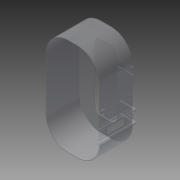
# Autodesk Inventor part: coil_former_mold_new
Saved by Autodesk Inventor 2014 SP1 (Build 180222100, 222)
## iProperties
Created: 2016-09-07
Part Number: coil_former_mold_new
Material: Polycarbonate, Clear
Document SubType Name: Modeling
Designer: tguillod
Density: 1.2 g/cm^3
Appearance: Polycarbonate - Clear
Author: tguillod
Autodesk Inventor part; units mm, degrees
ref_plane "YZ Plane" through (0, 0, 0) normal (1, 0, 0) x (0, 1, 0)
ref_plane "XZ Plane" through (0, 0, 0) normal (0, 1, 0) x (-1, 0, 0)
ref_plane "XY Plane" through (0, 0, 0) normal (0, 0, 1) x (1, 0, 0)
sketch "Sketch1" plane through (0, 0, 0) normal (0, 0, 1) x (1, 0, 0)
  line L0 (0, 0) -> (1, 0)
  line L1 (1, 0) -> (1, 57.5)
  line L2 (1, 57.5) -> (0, 57.5)
  line L3 (0, 57.5) -> (0, 0)
  line L4 (1, 57.5) -> (-26, 57.5)
  line L5 (-26, 57.5) -> (-26, 58.5)
  line L6 (-26, 58.5) -> (1, 58.5)
  line L7 (1, 58.5) -> (1, 57.5)
  dimension "d90" = 10
  dimension "d1" = 1
  dimension "d7" = 1
  dimension "d8" = 27
  dimension "d9" = 58.5
  constraints: 16 end point, 4 parallel, 2 horizontal, 2 perpendicular
  measures "d1" distance of L0.start L0.end
  measures "d7" distance of L6.end L1.end
  measures "d8" distance of L5.end L6.end
  measures "d9" distance from line of L0.end L6
sketch "Sketch2" plane through (0, 0, 0) normal (0, 1, 0) x (-1, 0, 0)
  line L0 (0, 0) -> (0, 46.75)
  line L1 (37, 83.75) -> (45.5, 83.75)
  arc A0 (37, 83.75) -> (0, 46.75) centre (37, 46.75) ccw
  point P0 (0, 83.75)
  dimension "d3" = 83.75
  dimension "d4" = 45.5
  dimension "d5" = 37
  constraints: 4 end point, 2 point on circle, 2 point on line, 2 tangent, 1 centre point, 1 perpendicular, 1 vertical
  measures "d3" distance of L0.start point (0, 83.75)
  measures "d4" distance of point (0, 83.75) L1.end
  measures "d5" radius of A0
sweep "Sweep1" add profiles "Sketch1" path "Sketch2" path curves L0 A0 L1
mirror "Mirror1" about plane through (0.5, 28.75, 0) normal (0, 0, -1)
mirror "Mirror2" about plane through (-45.5, 28.75, -84.25) normal (-1, 0, 0)
sketch "Sketch3" plane through (-26, 58.5, 0) normal (0, 1, 0) x (1, 0, 0)
  line L0 (27, 0) -> (0, 0) projected
  line L1 (0, 0) -> (0, -46.75) projected
  line L2 (0, -40) -> (10, -40)
  line L3 (10, -40) -> (10, -30)
  line L4 (10, -30) -> (0, -30)
  line L5 (0, -30) -> (0, -40)
  point P0 (26, 0)
  dimension "d10" = 30
  dimension "d11" = 10
  dimension "d12" = 10
  constraints: 8 end point, 2 parallel, 1 collinear, 1 horizontal, 1 perpendicular
  measures "d10" distance between parallel lines of L0 L4
  measures "d11" distance of L2.end L3.end
  measures "d12" distance of L2.start L2.end
extrude "Extrusion1" cut sketch "Sketch3" against normal blind 10
sketch "Sketch4" plane through (1, 58.5, 46.75) normal (0, 1, 0) x (1, 0, 0)
  line L0 (0, 93.5) -> (0, 0) projected
  line L1 (-7, 80.25) -> (-2, 80.25)
  line L2 (-2, 80.25) -> (-2, 76.25)
  line L3 (-2, 76.25) -> (-7, 76.25)
  line L4 (-7, 76.25) -> (-7, 80.25)
  point P0 (-1, 46.75)
  dimension "d16" = 5
  dimension "d17" = 4
  dimension "d18" = 2
  dimension "d19" = 29.5
  constraints: 8 end point, 2 parallel, 1 horizontal, 1 perpendicular
  measures "d16" distance of L1.start L1.end
  measures "d17" distance of L1.end L2.end
  measures "d18" distance between parallel lines of L0 L2
  measures "d19" distance from line of point (-1, 46.75) L3
extrude "Extrusion2" cut sketch "Sketch4" against normal blind 10
fillet "Fillet1" radius 3 2 edges at (-16, 58, 40) (-16, 58, 30)
sketch "Sketch7" plane through (1, 58.5, 46.75) normal (0, 1, 0) x (1, 0, 0)
  line L0 (-7, 80.25) -> (-2, 80.25) projected
  line L1 (-2, 76.25) -> (-7, 76.25) projected
  line L2 (-27, 93.5) -> (-27, 16.75) projected
  line L3 (0, 93.5) -> (0, 0) projected
  line L4 (-24, 88.25) -> (0, 88.25)
  line L5 (0, 88.25) -> (0, 87.25)
  line L6 (0, 87.25) -> (-24, 87.25)
  line L7 (-24, 87.25) -> (-24, 88.25)
  line L8 (0, 68.25) -> (-24, 68.25)
  line L9 (-24, 68.25) -> (-24, 69.25)
  line L10 (-24, 69.25) -> (0, 69.25)
  line L11 (0, 69.25) -> (0, 68.25)
  point P0 (-1, 46.75)
  dimension "d38" = 1
  dimension "d39" = 1
  dimension "d40" = 7
  dimension "d41" = 7
  dimension "d42" = 3
  constraints: 16 end point, 4 parallel, 2 horizontal, 2 perpendicular, 2 point on line, 1 collinear
  measures "d38" distance of L6.end L4.start
  measures "d39" distance of L8.end L9.end
  measures "d40" distance between parallel lines of L1 L10
  measures "d41" distance between parallel lines of L6 L0
  measures "d42" distance between parallel lines of L2 L7
extrude "Extrusion5" add sketch "Sketch7" along normal blind 3
sketch "Sketch8" plane through (1, 58.5, -41.5) normal (0, 0, -1) x (-1, 0, 0)
  line L0 (24, 0) -> (24, 3) projected
  line L1 (0, 3) -> (24, 3)
  line L2 (24, 3) -> (24, 2)
  line L3 (24, 2) -> (0, 2)
  line L4 (0, 2) -> (0, 3)
  point P0 (1, -58.5)
  dimension "d45" = 1
  constraints: 8 end point, 2 parallel, 1 horizontal, 1 perpendicular, 1 point on line
  measures "d45" distance of L1.end L2.end
extrude "Extrusion6" add sketch "Sketch8" along normal blind 1
sketch "Sketch9" plane through (-23, 58.5, -21.5) normal (0, 0, 1) x (1, 0, 0)
  line L0 (24, 0) -> (24, 3) projected
  line L1 (0, 3) -> (24, 3)
  line L2 (24, 3) -> (24, 2)
  line L3 (24, 2) -> (0, 2)
  line L4 (0, 2) -> (0, 3)
  point P0 (23, -58.5)
  dimension "d48" = 1
  constraints: 8 end point, 2 parallel, 1 horizontal, 1 perpendicular, 1 point on line
  measures "d48" distance of L1.end L2.end
extrude "Extrusion7" add sketch "Sketch9" along normal blind 1
sketch "Sketch10" plane through (1, 0, 46.75) normal (1, 0, 0) x (0, 0, -1)
  line L0 (68.25, 58.5) -> (68.25, 60.5) projected
  line L1 (93.5, 0) -> (0, 0) projected
  line L2 (69.25, 61.5) -> (68.25, 61.5)
  line L3 (68.25, 61.5) -> (68.25, -4)
  line L4 (68.25, -4) -> (69.25, -4)
  line L5 (69.25, -4) -> (69.25, 61.5)
  line L6 (87.25, 61.5) -> (88.25, 61.5)
  line L7 (88.25, 61.5) -> (88.25, -4)
  line L8 (88.25, -4) -> (87.25, -4)
  line L9 (87.25, -4) -> (87.25, 61.5)
  point P0 (88.25, 60.5)
  point P1 (46.75, 0)
  dimension "d51" = 4
  constraints: 16 end point, 4 parallel, 2 collinear, 2 horizontal, 2 perpendicular, 2 point on line
  measures "d51" distance between parallel lines of L1 L4
extrude "Extrusion8" add sketch "Sketch10" along normal blind 3
sketch "Sketch12" plane through (-23, 58.5, -21.5) normal (0, 0, 1) x (1, 0, 0)
  line L0 (24, -58.5) -> (24, -62.5) projected
  line L1 (24, -62.5) -> (27, -62.5) projected
  line L2 (27, 3) -> (27, -62.5) projected
  line L3 (24, 3) -> (27, 3) projected
  line L4 (24, 2) -> (24, 3) projected
  line L5 (24, -62.5) -> (24, -61.5)
  line L6 (26, -61.5) -> (26, 2)
  line L7 (26, 2) -> (24, 2)
  line L8 (24, 3) -> (27, 3)
  line L9 (27, -62.5) -> (27, 3)
  line L10 (27, -62.5) -> (24, -62.5)
  line L11 (24, -61.5) -> (26, -61.5)
  point P0 (23, -58.5)
  dimension "d56" = 1
  dimension "d57" = 1
  constraints: 14 end point, 3 collinear, 2 parallel, 1 perpendicular, 1 point on line
  measures "d56" distance between parallel lines of L9 L6
  measures "d57" distance between parallel lines of L1 L11
extrude "Extrusion9" add sketch "Sketch12" along normal blind 1
sketch "Sketch13" plane through (1, 58.5, -41.5) normal (0, 0, -1) x (-1, 0, 0)
  line L0 (24, 2) -> (0, 2) projected
  line L1 (0, 3) -> (0, 2) projected
  line L2 (0, 3) -> (-3, 3) projected
  line L3 (-3, -62.5) -> (-3, 3) projected
  line L4 (0, -62.5) -> (-3, -62.5) projected
  line L5 (0, -62.5) -> (0, -58.5) projected
  line L6 (24, 0) -> (0, 0) projected
  line L7 (0, 2) -> (0, 3)
  line L8 (-3, 3) -> (0, 3)
  line L9 (-3, 3) -> (-3, -62.5)
  line L10 (-3, -62.5) -> (0, -62.5)
  line L11 (0, -62.5) -> (0, -61.5)
  line L12 (-2, -61.5) -> (0, -61.5)
  line L13 (-2, -61.5) -> (-2, 2)
  line L14 (-2, 2) -> (0, 2)
  point P0 (1, -58.5)
  dimension "d60" = 1
  dimension "d61" = 1
  constraints: 16 end point, 4 perpendicular, 3 collinear, 1 point on line
  measures "d60" distance between parallel lines of L10 L12
  measures "d61" distance between parallel lines of L3 L13
extrude "Extrusion10" add sketch "Sketch13" along normal blind 1
sketch "Sketch16" plane through (1, 58.5, -22.5) normal (1, 0, 0) x (0, 0, -1)
  line L0 (0, 0) -> (0, -58.5) projected
  line L1 (18, -58.5) -> (0, -58.5) projected
  line L2 (18, -58.5) -> (18, 0) projected
  line L3 (18, 0) -> (0, 0) projected
  line L4 (3, 0) -> (4, 0)
  line L5 (4, 0) -> (4, -12)
  line L6 (4, -12) -> (3, -12)
  line L7 (3, -12) -> (3, 0)
  line L8 (15, 0) -> (14, 0)
  line L9 (14, 0) -> (14, -12)
  line L10 (14, -12) -> (15, -12)
  line L11 (15, -12) -> (15, 0)
  line L12 (3, -58.5) -> (4, -58.5)
  line L13 (4, -58.5) -> (4, -47.5)
  line L14 (4, -47.5) -> (3, -47.5)
  line L15 (3, -47.5) -> (3, -58.5)
  line L16 (15, -58.5) -> (14, -58.5)
  line L17 (14, -58.5) -> (14, -47.5)
  line L18 (14, -47.5) -> (15, -47.5)
  line L19 (15, -47.5) -> (15, -58.5)
  line L20 (3, -12) -> (15, -12)
  line L21 (15, -12) -> (15, -13)
  line L22 (15, -13) -> (3, -13)
  line L23 (3, -13) -> (3, -12)
  line L24 (3, -47.5) -> (15, -47.5)
  line L25 (15, -47.5) -> (15, -46.5)
  line L26 (15, -46.5) -> (3, -46.5)
  line L27 (3, -46.5) -> (3, -47.5)
  point P0 (-22.5, -58.5)
  dimension "d77" = 1
  dimension "d78" = 1
  dimension "d79" = 12
  dimension "d80" = 11
  dimension "d81" = 1
  dimension "d82" = 1
  dimension "d83" = 1
  dimension "d84" = 1
  dimension "d85" = 3
  dimension "d86" = 3
  dimension "d87" = 10
  dimension "d88" = 3
  dimension "d89" = 3
  dimension "d90" = 10
  constraints: 48 end point, 12 parallel, 6 horizontal, 6 perpendicular, 4 collinear, 4 point on line
  measures "d77" distance of L5.end L6.end
  measures "d78" distance of L9.end L10.end
  measures "d79" distance of L10.end L8.start
  measures "d80" distance of L18.end L16.start
  measures "d81" distance of L17.end L18.end
  measures "d82" distance of L13.end L14.end
  measures "d83" distance of L26.end L14.end
  measures "d84" distance of L22.end L6.end
  measures "d85" distance between parallel lines of L0 L7
  measures "d86" distance between parallel lines of L11 L2
  measures "d87" distance between parallel lines of L9 L5
  measures "d88" distance between parallel lines of L0 L15
  measures "d89" distance between parallel lines of L19 L2
  measures "d90" distance between parallel lines of L17 L13
extrude "Extrusion13" add sketch "Sketch16" along normal blind 1 contours L3 L5 L6 L7 | L15 L14 L13 L1 | L6 L20 L10 L21 L22 L23 | L27 L26 L25 L18 L24 L14 | L3 L11 L10 L9 | L17 L18 L19 L1
sketch "Sketch17" plane through (-54, 0, -84.75) normal (0, -1, 0) x (1, 0, 0)
  line L0 (56, 59.25) -> (55, 59.25)
  line L1 (55, 59.25) -> (55, 58.25)
  line L2 (55, 58.25) -> (56, 58.25)
  line L3 (56, 58.25) -> (56, 59.25)
  line L4 (56, 48.25) -> (55, 48.25)
  line L5 (55, 48.25) -> (55, 47.25)
  line L6 (55, 47.25) -> (56, 47.25)
  line L7 (56, 47.25) -> (56, 48.25)
  point P0 (54, 84.75)
  constraints: 16 end point, 4 parallel, 2 horizontal, 2 perpendicular
extrude "Extrusion14" add sketch "Sketch17" along normal blind 1
sketch "Sketch18" plane through (-54, 58.5, -84.75) normal (0, 1, 0) x (1, 0, 0)
  line L0 (55, -63.25) -> (55, -131.5) projected
  line L1 (28, -114.75) -> (55, -114.75)
  line L2 (55, -114.75) -> (55, -113.75)
  line L3 (55, -113.75) -> (28, -113.75)
  line L4 (28, -113.75) -> (28, -114.75)
  line L5 (28, -124.75) -> (55, -124.75)
  line L6 (55, -124.75) -> (55, -125.75)
  line L7 (55, -125.75) -> (28, -125.75)
  line L8 (28, -125.75) -> (28, -124.75)
  point P0 (54, -84.75)
  dimension "d95" = 1
  dimension "d96" = 1
  constraints: 16 end point, 4 parallel, 2 horizontal, 2 perpendicular, 2 point on line
  measures "d95" distance of L1.end L2.end
  measures "d96" distance between parallel lines of L5 L7
extrude "Extrusion15" add sketch "Sketch18" along normal blind 1
sketch "Sketch20" plane through (1, 0, 46.75) normal (1, 0, 0) x (0, 0, -1)
  line L0 (68.25, 58.5) -> (17.75, 58.5) projected
  line L1 (0, 0) -> (0, 58.5) projected
  line L2 (68.25, 0) -> (0, 0) projected
  line L3 (42.75, 55.5) -> (50.75, 55.5)
  line L4 (50.75, 55.5) -> (50.75, 48.5)
  line L5 (50.75, 48.5) -> (42.75, 48.5)
  line L6 (42.75, 48.5) -> (42.75, 55.5)
  line L7 (42.75, 9) -> (50.75, 9)
  line L8 (50.75, 9) -> (50.75, 2)
  line L9 (50.75, 2) -> (42.75, 2)
  line L10 (42.75, 2) -> (42.75, 9)
  line L11 (43.75, 54.5) -> (49.75, 54.5)
  line L12 (49.75, 54.5) -> (49.75, 49.5)
  line L13 (49.75, 49.5) -> (43.75, 49.5)
  line L14 (43.75, 49.5) -> (43.75, 54.5)
  line L15 (43.75, 8) -> (49.75, 8)
  line L16 (49.75, 8) -> (49.75, 3)
  line L17 (49.75, 3) -> (43.75, 3)
  line L18 (43.75, 3) -> (43.75, 8)
  point P0 (46.75, 0)
  dimension "d112" = 8
  dimension "d113" = 7
  dimension "d114" = 7
  dimension "d116" = 2
  dimension "d117" = 3
  dimension "d118" = 42.75
  dimension "d119" = 1
  dimension "d120" = 1
  dimension "d121" = 1
  dimension "d122" = 1
  dimension "d123" = 1
  dimension "d124" = 1
  dimension "d125" = 1
  dimension "d126" = 1
  constraints: 32 end point, 8 parallel, 4 horizontal, 4 perpendicular, 2 collinear
  measures "d112" distance of L3.start L3.end
  measures "d113" distance of L3.end L4.end
  measures "d114" distance of L7.end L8.end
  measures "d116" distance between parallel lines of L2 L9
  measures "d117" distance between parallel lines of L0 L3
  measures "d118" distance between parallel lines of L1 L6
  measures "d119" distance between parallel lines of L3 L11
  measures "d120" distance between parallel lines of L6 L14
  measures "d121" distance between parallel lines of L5 L13
  measures "d122" distance between parallel lines of L4 L12
  measures "d123" distance between parallel lines of L7 L15
  measures "d124" distance between parallel lines of L8 L16
  measures "d125" distance between parallel lines of L17 L9
  measures "d126" distance between parallel lines of L10 L18
extrude "Extrusion17" add sketch "Sketch20" along normal blind 1
fillet "Fillet7" radius 1 14 edges at (-45.5, 58.5, -84.75) (-80.8701, 58.5, -73.6201) (-92, 58.5, 0) (-80.8701, 58.5, 73.6201) (-45.5, 58.5, 84.75) (-10.1299, 58.5, 73.6201) (1, 58.5, 43.875) (1, 58.5, -44.125) (-10.1299, 58.5, -73.6201) (1, 58.5, 35) (1, 58.5, 3.75) (1, 58.5, -24) (1, 58.5, -31.5) (1, 58.5, -39)
fillet "Fillet8" radius 1 4 edges at (3, 60.5, -42) (3, -3, -42) (3, 60.5, -21) (3, -3, -21)
sketch "Sketch23" plane through (1, 0, 46.75) normal (-1, 0, 0) x (0, 0, 1)
  line L0 (-88.25, 0) -> (-87.25, 0) projected
  line L1 (-88.25, -3) -> (-88.25, 0) projected
  line L2 (-88.25, -3) -> (-89.25, -3) projected
  line L3 (-89.25, -4) -> (-89.25, -3) projected
  line L4 (-87.25, -4) -> (-89.25, -4) projected
  line L5 (-87.25, 0) -> (-87.25, -4) projected
  line L6 (-69.25, 0) -> (-68.25, 0) projected
  line L7 (-69.25, -4) -> (-69.25, 0) projected
  line L8 (-69.25, -4) -> (-67.25, -4) projected
  line L9 (-67.25, -3) -> (-67.25, -4) projected
  line L10 (-68.25, -3) -> (-67.25, -3) projected
  line L11 (-68.25, 0) -> (-68.25, -3) projected
  line L12 (-89.25, -3) -> (-87.25, -3)
  line L13 (-87.25, -3) -> (-87.25, -4)
  line L14 (-87.25, -4) -> (-89.25, -4)
  line L15 (-89.25, -4) -> (-89.25, -3)
  line L16 (-87.25, -3) -> (-88.25, -3)
  line L17 (-88.25, -3) -> (-88.25, 0)
  line L18 (-88.25, 0) -> (-87.25, 0)
  line L19 (-87.25, 0) -> (-87.25, -3)
  line L20 (-88.25, 0) -> (-89.25, 0)
  line L21 (-89.25, 0) -> (-89.25, -1)
  line L22 (-89.25, -1) -> (-88.25, -1)
  line L23 (-88.25, -1) -> (-88.25, 0)
  line L24 (-67.25, -3) -> (-69.25, -3)
  line L25 (-69.25, -3) -> (-69.25, -4)
  line L26 (-69.25, -4) -> (-67.25, -4)
  line L27 (-67.25, -4) -> (-67.25, -3)
  line L28 (-68.25, -3) -> (-69.25, -3)
  line L29 (-69.25, -3) -> (-69.25, 0)
  line L30 (-69.25, 0) -> (-68.25, 0)
  line L31 (-68.25, 0) -> (-68.25, -3)
  line L32 (-68.25, 0) -> (-67.25, 0)
  line L33 (-67.25, 0) -> (-67.25, -1)
  line L34 (-67.25, -1) -> (-68.25, -1)
  line L35 (-68.25, -1) -> (-68.25, 0)
  point P0 (-46.75, 0)
  constraints: 48 end point, 12 parallel, 6 horizontal, 6 perpendicular, 4 collinear
extrude "Extrusion19" add sketch "Sketch23" along normal blind 2
fillet "Fillet10" radius 1 2 edges at (1, -1, -42) (1, -1, -21)
fillet "Fillet11" radius 1 20 edges at (-0.5, -1, -41.5) (1, 28.75, -41.5) (0.7071, 58.2071, -41.5) (-11.5, 58.5, -41.5) (0.7071, -0.7071, -41.5) (2.7071, -2.7071, -41.5) (3, 28.75, -41.5) (2.7071, 60.2071, -41.5) (-10.5, 60.5, -41.5) (0.5, -3, -41.5) (2.7071, -2.7071, -21.5) (3, 28.75, -21.5) (2.7071, 60.2071, -21.5) (-10.5, 60.5, -21.5) (0.5, -3, -21.5) (1, 28.75, -21.5) (0.7071, 58.2071, -21.5) (-11.5, 58.5, -21.5) (-0.5, -1, -21.5) (0.7071, -0.7071, -21.5)
sketch "Sketch24" plane through (0, 0, -42.5) normal (0, 0, -1) x (-1, 0, 0)
  line L0 (23, 60.5) -> (23, 61.5) projected
  line L1 (23, 61.5) -> (-4, 61.5) projected
  line L2 (-4, 61.5) -> (-4, -4) projected
  line L3 (-4, -4) -> (1, -4) projected
  line L4 (1, -3) -> (1, -4) projected
  line L5 (-2, -3) -> (1, -3) projected
  arc A0 (-3, -2) -> (-2, -3) centre (-2, -2) ccw projected
  line L6 (-3, -2) -> (-3, 59.5) projected
  arc A1 (-2, 60.5) -> (-3, 59.5) centre (-2, 59.5) ccw projected
  line L7 (-2, 60.5) -> (23, 60.5) projected
  line L8 (1, 0) -> (-1, 0)
  line L9 (-1, 0) -> (-1, -4)
  line L10 (-1, -4) -> (1, -4)
  line L11 (1, -4) -> (1, 0)
  constraints: 8 end point, 2 parallel, 1 horizontal, 1 perpendicular, 1 point on line
extrude "Extrusion20" cut sketch "Sketch24" against normal through all contours L9 L5 L4 L3 | L9 L8 L11 L5
sketch "Sketch25" plane through (1, 45.5, -25.5) normal (1, 0, 0) x (0, 0, -1)
  line L0 (12, 0) -> (0, 0) projected
  line L1 (-3, 12) -> (-3, -45.5) projected
  line L2 (0, -33.5) -> (12, -33.5) projected
  line L3 (15, -45.5) -> (15, 12) projected
  line L4 (1, -2) -> (11, -2)
  line L5 (11, -2) -> (11, -31.5)
  line L6 (11, -31.5) -> (1, -31.5)
  line L7 (1, -31.5) -> (1, -2)
  point P0 (-25.5, -45.5)
  dimension "d145" = 2
  dimension "d146" = 2
  dimension "d147" = 4
  dimension "d148" = 4
  constraints: 8 end point, 2 parallel, 1 horizontal, 1 perpendicular
  measures "d145" distance between parallel lines of L0 L4
  measures "d146" distance between parallel lines of L2 L6
  measures "d147" distance between parallel lines of L1 L7
  measures "d148" distance between parallel lines of L5 L3
extrude "Extrusion21" cut sketch "Sketch25" against normal blind 10
sketch "Sketch27" plane through (1, 45.5, -25.5) normal (1, 0, 0) x (0, 0, -1)
  line L0 (12, 12) -> (15, 12) projected
  line L1 (-3, 12) -> (0, 12) projected
  line L2 (0, -45.5) -> (-3, -45.5) projected
  line L3 (15, -45.5) -> (12, -45.5) projected
  line L4 (-7, 12) -> (-8, 12)
  line L5 (-8, 12) -> (-8, -45.5)
  line L6 (-8, -45.5) -> (-7, -45.5)
  line L7 (-7, -45.5) -> (-7, 12)
  line L8 (19, 12) -> (20, 12)
  line L9 (20, 12) -> (20, -45.5)
  line L10 (20, -45.5) -> (19, -45.5)
  line L11 (19, -45.5) -> (19, 12)
  line L12 (-5, -49.5) -> (-5, 16) projected
  line L13 (17, 16) -> (17, -49.5) projected
  point P0 (-25.5, -45.5)
  dimension "d151" = 1
  dimension "d152" = 1
  dimension "d153" = 2
  dimension "d154" = 2
  constraints: 16 end point, 4 collinear, 4 parallel, 2 horizontal, 2 perpendicular
  measures "d151" distance of L4.start L4.end
  measures "d152" distance of L8.start L8.end
  measures "d153" distance between parallel lines of L7 L12
  measures "d154" distance between parallel lines of L11 L13
extrude "Extrusion22" add sketch "Sketch27" along normal blind 1
body "Solid1"
